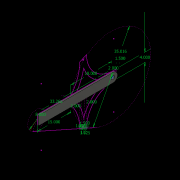
# Autodesk Inventor part: 250_Neck
Saved by Autodesk Inventor 2021 (Build 250183000, 183)
## iProperties
Created: 2020-11-11
Part Number: 250_Neck
Material: Steel
Document SubType Name: Modeling
Designer: Dylan
Density: 7.85 g/cm^3
Appearance: Plate
Mass: 11436.9 g
Surface Area: 1915.28 cm^2
Volume: 1456.93 cm^3
Author: Dylan
Autodesk Inventor part; units mm, degrees
ref_plane "YZ Plane" through (0, 0, 0) normal (1, 0, 0) x (0, 1, 0)
ref_plane "XZ Plane" through (0, 0, 0) normal (0, 1, 0) x (-1, 0, 0)
ref_plane "XY Plane" through (0, 0, 0) normal (0, 0, 1) x (1, 0, 0)
sketch "Sketch1" plane through (0, 0, 0) normal (1, 0, 0) x (0, 1, 0)
  line L0 (0, 0) -> (101.6, 0)
  line L1 (101.6, 0) -> (101.6, -508)
  line L2 (101.6, -508) -> (0, -508)
  line L3 (0, -508) -> (0, 0)
  circle A0 centre (50.8, -457.2) radius 19.05
  line L4 (50.8, 0) -> (50.8, -508) construction
  line L5 (101.6, -457.2) -> (0, -457.2) construction
  circle A1 centre (50.8, -457.2) radius 19.05
  circle A2 centre (50.8, -457.2) radius 444.7032 construction
  line L6 (-355.5868, -276.6157) -> (-378.1625, -327.4201) construction
  circle A3 centre (50.8, 387.719) radius 101.6 construction
  line L7 (50.8, 387.719) -> (-21.056, 459.5471) construction
  line L8 (44.4149, -276.5368) -> (44.4051, -225.7368) construction
  line L9 (50.8, 387.719) -> (50.8197, 286.119) construction
  line L10 (-42.046, 428.9765) -> (-355.5868, -276.6157)
  circle A4 centre (-277.7933, -136.7333) radius 14.2875 construction
  line L11 (50.8, 387.719) -> (50.8, -457.2) construction
  circle A5 centre (-277.7933, -136.7333) radius 6.35
  line L12 (-277.7933, -136.7333) -> (-290.8498, -130.9315) construction
  line L13 (-283.5962, -134.1547) -> (-290.8498, -130.9315) construction
  line L14 (-290.8498, -130.9315) -> (-288.9928, -131.7566) construction
  line L15 (-277.7933, -136.7333) -> (-277.7933, -151.0208) construction
  line L16 (-277.7933, -136.7333) -> (-263.5058, -136.7333) construction
  line L17 (-277.7933, -136.7333) -> (-277.7933, -122.4458) construction
  line L18 (-277.7933, -122.4458) -> (0, -122.4458) construction
  line L19 (-277.7933, -151.0208) -> (0, -151.0208) construction
  line L20 (-277.7933, -122.4458) -> (-288.3972, -146.3088) construction
  line L21 (-288.9928, -131.7566) -> (-308.1346, -174.8333)
  line L22 (-288.9928, -131.7566) -> (-274.274, -98.6333)
  line L23 (-308.1346, -174.8333) -> (0, -174.8333) construction
  line L24 (-274.274, -98.6333) -> (0, -98.6333) construction
  arc A6 (-274.274, -98.6333) -> (0, 0) centre (-274.274, 332.0263) ccw
  circle A7 centre (50.8, -457.2) radius 50.8
  arc A8 (0, -457.2) -> (-308.1346, -174.8333) centre (-308.1346, -484.1437) ccw
  arc A9 (22.8389, -342.2423) -> (-308.1346, -124.0333) centre (-308.1346, -484.1437) ccw construction
  arc A10 (-274.274, -149.4333) -> (157.8944, 119.8146) centre (-274.274, 332.0263) ccw construction
  arc A11 (0, -297.777) -> (-193.8113, -142.6621) centre (-308.1346, -484.1437) ccw
  arc A12 (-193.8113, -142.6621) -> (0, -63.672) centre (-274.274, 332.0263) ccw
  line L25 (101.6, -508) -> (101.6, 0)
  circle A13 centre (379.3933, -136.7333) radius 6.35
  line L26 (390.5928, -131.7566) -> (409.7346, -174.8333)
  line L27 (390.5928, -131.7566) -> (375.874, -98.6333)
  arc A14 (101.6, 0) -> (375.874, -98.6333) centre (375.874, 332.0263) ccw
  arc A15 (409.7346, -174.8333) -> (101.6, -457.2) centre (409.7346, -484.1437) ccw
  arc A16 (295.4113, -142.6621) -> (101.6, -297.777) centre (409.7346, -484.1437) ccw
  arc A17 (101.6, -63.672) -> (295.4113, -142.6621) centre (375.874, 332.0263) ccw
  line L28 (101.6, 0) -> (0, 0)
  line L29 (0, 0) -> (0, 381)
  line L30 (0, 381) -> (101.6, 381)
  line L31 (101.6, 381) -> (101.6, 0)
  line L32 (50.8, 387.719) -> (-42.046, 428.9765) construction
  point P0 (101.6, -63.672)
  point P1 (101.6, -297.777)
  dimension "d11" = 889.4064
  dimension "d18" = 12.7
  dimension "d0" = 101.6
  dimension "d2" = 50.8
  dimension "d3" = 38.1
  dimension "d16" = 28.575
  dimension "d17" = 203.2
  dimension "d19" = 2.032
  dimension "d20" = 90
  dimension "d23" = 38.1
  dimension "d24" = 38.1
  dimension "d25" = 844.919
  dimension "d28" = 50.8
  dimension "d29" = 50.8
  dimension "d30" = 457.2
  dimension "d32" = 381
  constraints: 64 end point, 30 point on circle, 15 centre point, 11 symmetric about line, 8 horizontal, 8 point on line, 6 parallel, 5 tangent, 4 coincident, 4 midpoint, 3 concentric, 2 equal length, 2 perpendicular, 1 collinear, 1 vertical, 27 other
  measures "d0" distance of L1.end L2.end
  measures "d2" distance between parallel lines of L2 L5
  measures "d3" diameter of A0
  measures "d16" diameter of A4
  measures "d17" diameter of A3
  measures "d19" distance of L12.end L14.end
  measures "d20" angle of L15 L16
  measures "d23" distance from line of L23 A4.centre
  measures "d24" distance from line of L24 A4.centre
  measures "d25" distance of L9.start L11.end
  measures "d28" radial gap between concentric circles of A8 A9
  measures "d29" radial gap between concentric circles of A6 A10
  measures "d30" distance from line of L0 point (50.8, -457.2)
  measures "d32" distance of L28.end L29.end
extrude "Extrusion1" add sketch "Sketch1" along normal blind 19.05 contours L29 L30 L31 L0 | L0 L1 A7 L3 | A7
body "Solid1"
